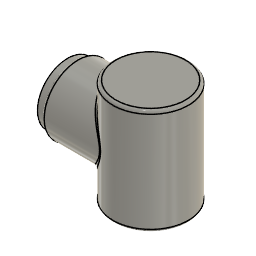
Assembly (Autodesk Fusion 360 archive; units mm, degrees)
design "link 04"
part number: 2026-05-23-14-39-53-080
Autodesk Fusion 360 part; units mm, degrees
note: some values were not read from the file. Set by a fixed rule: the direction of a hole.
sketch "Sketch1" plane through (0, 0, 0) normal (0, 0, 1) x (1, 0, 0)
  circle A0 centre (0, 0) radius 25
  dimension "d1" = 50
  constraint coincident A0.centre origin
  measures "d1" diameter of A0
extrude "Extrude1" add sketch "Sketch1" along normal blind 70
sketch "Sketch2" plane through (0, 0, 0) normal (1, 0, 0) x (0, 1, 0)
  circle A0 centre (0, 35) radius 22.5
  point P0 (0, 70)
  dimension "d4" = 45
  dimension "d5" = 35
  measures "d4" diameter of A0
  measures "d5" vertical distance of A0.centre P0
extrude "Extrude2" add sketch "Sketch2" against normal blind 50
sketch "Sketch3" plane through (-50, 0, 0) normal (-1, 0, 0) x (0, -1, 0)
sketch "Sketch4" plane through (-50, 0, 0) normal (-1, 0, 0) x (0, -1, 0)
sketch "Sketch5" plane through (-50, 0, 0) normal (-1, 0, 0) x (0, -1, 0)
  circle A0 centre (0, 35) radius 20
  dimension "d12" = 40
  measures "d12" diameter of A0
extrude "Extrude3" add sketch "Sketch5" along normal blind 5
fillet "Fillet3" radius 2 4 edges at (-23.3082, -9.0404, 70) (-23.3082, -9.0404, 0) (-10.8972, 22.5, 35) (-50, -20.9774, 43.1363)

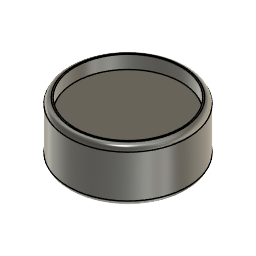
design "link 05"
part number: 2026-05-23-15-50-52-912
Autodesk Fusion 360 part; units mm, degrees
sketch "Sketch1" plane through (0, 0, 0) normal (0, 0, 1) x (1, 0, 0)
  circle A0 centre (0, 0) radius 22.5
  dimension "d1" = 45
  constraint coincident A0.centre origin
  measures "d1" diameter of A0
extrude "Extrude1" add sketch "Sketch1" along normal blind 20
sketch "Sketch2" plane through (0, 0, 20) normal (0, 0, 1) x (-1, 0, 0)
  circle A0 centre (0, 0) radius 22.5
  circle A1 centre (0, 0) radius 20
  dimension "d4" = 40
  constraint coincident A0.centre A1.centre
  measures "d4" diameter of A1
extrude "Extrude2" cut sketch "Sketch2" against normal blind 5 contours A1
sketch "Sketch3" plane through (0, 0, 0) normal (0, 0, 1) x (1, 0, 0)
  circle A0 centre (0, 0) radius 12.5
  dimension "d7" = 25
  constraint coincident A0.centre origin
  measures "d7" diameter of A0
extrude "Extrude3" cut sketch "Sketch3" along normal blind 5
sketch "Sketch4" plane through (0, 0, 0) normal (0, 0, -1) x (1, 0, 0)
  circle A0 centre (0, 0) radius 12.5
  circle A1 centre (0, 0) radius 22.5
  circle A2 centre (0, 0) radius 17.2047
  line L0 (0, 0) -> (-12, 12)
  line L1 (-12, 12) -> (0, 0)
  line L2 (0, 0) -> (12.1655, -12.1655)
  line L3 (0, 0) -> (12, 12)
  line L4 (12, 12) -> (0, 0)
  line L5 (0, 0) -> (-12, -12)
  point P0 (0, 17.2047)
  point P1 (12.1655, 12.1655)
  point P2 (17.2045, -0.0657)
  point P3 (12.1655, -12.1655)
  point P4 (-0.0267, -17.2046)
  point P5 (-12.1655, -12.1655)
  point P6 (-12, 12)
  point P7 (-17.2047, 0)
  constraint coincident A0.centre A1.centre
  constraint coincident A2 P0
  constraint coincident A2 P3
  constraint parallel L1 L2
  constraint perpendicular L2 L3
  constraint perpendicular L1 L5
  constraint coincident A2 P1
  constraint coincident A2 P2
  constraint coincident P3 L2.end
  constraint coincident A2 P4
  constraint coincident A2 P5
  constraint coincident P6 L0.end
  constraint coincident A2 P7
hole "Hole1" at (0, -17.2047, 0) at (-12, -12, 0) at (-17.2047, 0, 0) at (-12, 12, 0) at (-0.0267, 17.2046, 0) at (12.1655, 12.1655, 0) at (17.2045, 0.0657, 0) at (12.1655, -12.1655, 0) direction (0, 0, 1) diameter 5.035 depth 6 tip angle 118
thread "Thread1" "ISO Metric profile 6.0 M6x1 M6x1 6H" thread offset 0 thread depth 7.4
fillet "Fillet1" radius 2 1 edges at (-20.9774, -8.1363, 20) 1 faces at (-22.472, 1.1215, 6.6667)

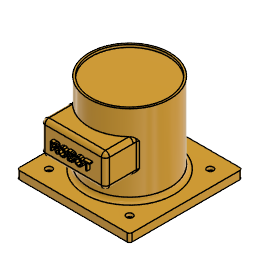
design "base"
part number: 2026-05-23-09-46-44-158
Autodesk Fusion 360 part; units mm, degrees
sketch "Sketch1" plane through (0, 0, 0) normal (0, 0, 1) x (1, 0, 0)
  line L0 (-70, 70) -> (70, 70)
  line L1 (70, 70) -> (70, -70)
  line L2 (70, -70) -> (-70, -70)
  line L3 (-70, -70) -> (-70, 70)
  constraint horizontal L0
  constraint vertical L1
  constraint horizontal L2
  constraint vertical L3
extrude "Extrude1" add sketch "Sketch1" along normal blind 10
sketch "Sketch2" plane through (0, 0, 10) normal (0, 0, 1) x (-1, 0, 0)
  line L0 (70, 70) -> (-70, 70)
  line L1 (-70, 70) -> (-70, -70)
  line L2 (-70, -70) -> (70, -70)
  line L3 (70, -70) -> (70, 70)
  circle A0 centre (0, 0) radius 50
  dimension "d3" = 100
  constraint coincident A0.centre origin
  measures "d3" diameter of A0
extrude "Extrude2" add sketch "Sketch2" along normal blind 100 contours A0
sketch "Sketch3" plane through (0, 0, 0) normal (0, 1, 0) x (1, 0, 0)
  line L0 (-40, -80) -> (40, -80)
  line L1 (40, -80) -> (40, -40)
  line L2 (40, -40) -> (-40, -40)
  line L3 (-40, -40) -> (-40, -80)
  dimension "d6" = 80
  dimension "d7" = 40
  dimension "d8" = 40
  dimension "d9" = 40
  constraint horizontal L0
  constraint vertical L1
  constraint horizontal L2
  constraint vertical L3
  measures "d6" distance of L0.start L0.end
  measures "d7" distance of L0.start L2.end
  measures "d8" horizontal distance of origin L2.end
  measures "d9" distance of origin L2
extrude "Extrude3" add sketch "Sketch3" against normal blind 70
sketch "Sketch4" plane through (0, 0, 110) normal (0, 0, 1) x (-1, 0, 0)
  circle A0 centre (0, 0) radius 50
  circle A1 centre (0, 0) radius 47.5
  dimension "d12" = 95
  constraint coincident A0.centre A1.centre
  measures "d12" diameter of A1
extrude "Extrude4" cut sketch "Sketch4" against normal blind 3 contours A1
sketch "Sketch5" plane through (0, 0, 10) normal (0, 0, 1) x (-1, 0, 0)
  circle A0 centre (0, 0) radius 50
  line L0 (70, 70) -> (-70, 70)
  line L1 (-70, 70) -> (-70, -70)
  line L2 (-70, -70) -> (70, -70)
  line L3 (70, -70) -> (70, 70)
  point P0 (50, -50)
  point P1 (-50, -50)
  point P2 (-50, 50)
  point P3 (50, 50)
  dimension "d15" = 20
  dimension "d16" = 20
  dimension "d17" = 20
  dimension "d18" = 20
  dimension "d19" = 20
  dimension "d20" = 20
  dimension "d21" = 20
  dimension "d22" = 20
  measures "d15" vertical distance of L2.end P0
  measures "d16" horizontal distance of L2.end P0
  measures "d17" vertical distance of L1.end P1
  measures "d18" horizontal distance of L1.end P1
  measures "d19" vertical distance of L0.end P2
  measures "d20" horizontal distance of L0.end P2
  measures "d21" vertical distance of L0.start P3
  measures "d22" horizontal distance of L0.start P3
hole "Hole1" at (50, 50, 10) at (-50, 50, 10) at (-50, -50, 10) at (50, -50, 10) direction (0, 0, -1) diameter 4.5 depth 40 tip angle 118 counterbore diameter 8 counterbore depth 4
fillet "Fillet1" radius 3 4 edges at (70, -70, 5) (-70, -70, 5) (70, 70, 5) (-70, 70, 5)
fillet "Fillet2" radius 5 4 edges at (40, -70, 60) (-40, -70, 60) (-40, -30, 60) (40, -30, 60)
fillet "Fillet3" radius 5 7 edges at (40.2327, -30.1152, 80) (40, -48.3114, 80) (38.5355, -68.5355, 80) (0, -70, 80) (-38.5355, -68.5355, 80) (-40, -48.3114, 80) (-40.2327, -30.1152, 80)
fillet "Fillet4" radius 5 7 edges at (-40.2327, -30.1152, 40) (-40, -48.3114, 40) (-38.5355, -68.5355, 40) (0, -70, 40) (38.5355, -68.5355, 40) (40, -48.3114, 40) (40.2327, -30.1152, 40)
fillet "Fillet5" radius 5 1 edges at (46.6164, -18.0808, 10)
sketch "Sketch7" plane through (0, -70, 0) normal (0, -1, 0) x (1, 0, 0)
  line L0 (-35, 45) -> (35, 45)
  line L1 (35, 45) -> (35, 75)
  line L2 (35, 75) -> (-35, 75)
  line L3 (-35, 75) -> (-35, 45)
  line L4 (-35, 45) -> (35, 45) construction
  line L5 (35, 45) -> (35, 75) construction
  line L6 (35, 75) -> (-35, 75) construction
  line L7 (-35, 75) -> (-35, 45) construction
  dimension "d44" = 10
  text T0 "ROBOT" font "Arial" height 10 align centre middle in box 70 x 30 at (-35, 45) x (1, 0) y (0, 1) spacing 1 kerned
  constraint coincident L0.end
  constraint coincident L2.end
extrude "Extrude6" add sketch "Sketch7" along normal blind 4 text T0
equation "d45 = 'ROBOT'"

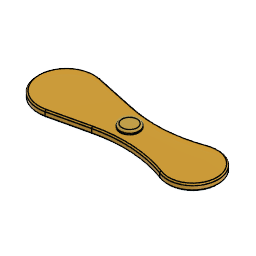
design "Link 01"
part number: 2026-05-23-11-57-22-292
Autodesk Fusion 360 part; units mm, degrees
sketch "Sketch1" plane through (0, 0, 0) normal (0, 0, 1) x (1, 0, 0)
  circle A0 centre (0, 0) radius 45
  circle A1 centre (200, 0) radius 40
  line L0 (9.3968, 44.008) -> (75, 30)
  arc A2 (75, 30) -> (188.4082, 38.2835) centre (117.4765, 228.9292) ccw
  line L1 (10.1387, -43.843) -> (70, -30)
  arc A3 (184.6116, -36.9215) -> (70, -30) centre (115.6051, -227.2104) ccw
  dimension "d1" = 90
  dimension "d2" = 80
  dimension "d3" = 200
  constraint coincident A0.centre origin
  constraint coincident A0 L0.start
  constraint tangent A0 L0
  constraint coincident A1 A2.end
  constraint tangent L0 A2
  constraint coincident A0 L1.start
  constraint tangent A0 L1
  constraint coincident A1 A3.start
  constraint tangent L1 A3
  measures "d1" diameter of A0
  measures "d2" diameter of A1
  measures "d3" distance of A0.centre A1.centre
extrude "Extrude1" add sketch "Sketch1" along normal blind 10
sketch "Sketch3" plane through (0, 0, 0) normal (0, 0, -1) x (1, 0, 0)
  arc A0 (10.1387, 43.843) -> (9.3968, -44.008) centre (0, 0) ccw
  line L0 (9.3968, -44.008) -> (75, -30)
  arc A1 (184.4992, -36.8744) -> (75, -30) centre (117.4765, -228.9292) ccw
  arc A2 (184.4992, -36.8744) -> (184.6116, 36.9215) centre (200, 0) ccw
  arc A3 (70, 30) -> (184.6116, 36.9215) centre (115.6051, 227.2104) ccw
  line L1 (70, 30) -> (10.1387, 43.843)
fillet "Fillet3" radius 2 12 edges at (130.2218, 25.9153, 10) (42.1984, 37.004, 10) (-44.9984, -0.38, 10) (40.0694, -36.9215, 10) (127.8069, -25.1637, 10) (240, 0.0609, 10) (240, 0.0609, 0) (127.8069, -25.1637, 0) (40.0694, -36.9215, 0) (-44.9984, -0.38, 0) (42.1984, 37.004, 0) (130.2218, 25.9153, 0)
sketch "Sketch4" plane through (0, 0, 10) normal (0, 0, 1) x (-1, 0, 0)
  arc A0 (-185.3383, 35.0576) -> (-185.2178, -35.0069) centre (-200, 0) ccw
  arc A1 (-74.5824, -28.0441) -> (-185.2178, -35.0069) centre (-117.4765, -228.9292) ccw
  line L0 (-74.5824, -28.0441) -> (-8.9792, -42.052)
  arc A2 (-8.9792, -42.052) -> (-9.6881, 41.8944) centre (0, 0) ccw
  line L1 (-9.6881, 41.8944) -> (-69.5494, 28.0514)
  arc A3 (-185.3383, 35.0576) -> (-69.5494, 28.0514) centre (-115.6051, 227.2104) ccw
  circle A4 centre (-100, 0) radius 15
  dimension "d22" = 30
  measures "d22" diameter of A4
extrude "Extrude2" add sketch "Sketch4" along normal blind 5 contours A4
sketch "Sketch5" plane through (0, 0, 15) normal (0, 0, 1) x (-1, 0, 0)
  circle A0 centre (-100, 0) radius 15
fillet "Fillet4" radius 3 1 faces at (105.2189, -1.9491, 15)

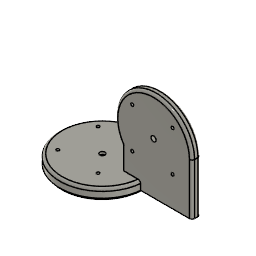
design "Link"
part number: 2026-05-23-10-24-38-964
Autodesk Fusion 360 part; units mm, degrees
sketch "Sketch1" plane through (0, 0, 0) normal (0, 0, 1) x (1, 0, 0)
sketch "Sketch2" plane through (0, 0, 0) normal (0, 0, 1) x (1, 0, 0)
sketch "Sketch3" plane through (0, 0, 0) normal (0, 0, 1) x (1, 0, 0)
sketch "Sketch4" plane through (0, 0, 0) normal (0, 0, 1) x (1, 0, 0)
  circle A0 centre (0, 0) radius 50
  dimension "d1" = 100
  constraint coincident A0.centre origin
  measures "d1" diameter of A0
extrude "Extrude1" add sketch "Sketch4" along normal blind 10
sketch "Sketch5" plane through (0, 0, 0) normal (0, 0, 1) x (1, 0, 0)
  circle A0 centre (0, 0) radius 47.5
  dimension "d4" = 95
  constraint coincident A0.centre origin
  measures "d4" diameter of A0
extrude "Extrude2" add sketch "Sketch5" against normal blind 3
sketch "Sketch6" plane through (0, 0, 0) normal (0, 1, 0) x (1, 0, 0)
  line L0 (30, 0) -> (110, 0)
  line L1 (110, 0) -> (110, -50)
  line L2 (110, -50) -> (110, -60)
  arc A0 (30, -31.7157) -> (110, -60) centre (65, -60) ccw
  line L3 (30, -31.7157) -> (30, 0)
  dimension "d7" = 80
  dimension "d8" = 50
  dimension "d9" = 45
  dimension "d10" = 30
  dimension "d11" = 60
  constraint horizontal L0
  constraint perpendicular L0 L1
  constraint parallel L1 L2
  constraint tangent L2 A0
  constraint perpendicular L0 L3
  measures "d7" distance of L0.start L0.end
  measures "d8" distance of L0.end L1.end
  measures "d9" radius of A0
  measures "d10" distance of origin L0.start
  measures "d11" vertical distance of origin A0.centre
extrude "Extrude3" add sketch "Sketch6" along normal mid plane 10
sketch "Sketch7" plane through (0, 5, 0) normal (0, 1, 0) x (-1, 0, 0)
  line L0 (-49.7494, 10) -> (-30, 10)
  line L1 (-30, 10) -> (-30, 31.7157)
  arc A0 (-30, 31.7157) -> (-110, 60) centre (-65, 60) ccw
  line L2 (-110, 60) -> (-110, 0)
  line L3 (-110, 0) -> (-49.7494, 0)
  line L4 (-49.7494, 0) -> (-49.7494, 10)
  line L5 (-87.244, 82.244) -> (-40, 82.244)
  line L6 (-40, 82.244) -> (-40, 35)
  line L7 (-40, 35) -> (-87.244, 35)
  line L8 (-87.244, 35) -> (-87.244, 82.244)
  dimension "d14" = 47.244
  dimension "d15" = 47.244
  dimension "d16" = 25
  dimension "d17" = 25
  constraint horizontal L5
  constraint vertical L6
  constraint horizontal L7
  constraint vertical L8
  measures "d14" distance of L5.start L5.end
  measures "d15" distance of L5.start L7.end
  measures "d16" vertical distance of A0.centre L7.end
  measures "d17" horizontal distance of A0.centre L6.end
hole "Hole1" at (40, 5, 82.244) at (87.244, 5, 82.244) at (87.244, 5, 35) at (40, 5, 35) direction (0, -1, 0) diameter 3.332 end through all
thread "Thread2" "ISO Metric profile 4.0 M4x0.7 M4x0.7 6H" major diameter 4.1095 minor diameter 3.332 pitch 0.7 angle 60 resizes the face on face at (39.2032, 1.6667, 33.5369) on face at (88.4931, 1.6667, 33.8976) on face at (38.3345, 1.6667, 82.2025) on face at (85.9949, 1.6667, 83.3464)
hole "Hole2" at (65, 5, 60) direction (0, -1, 0) diameter 6 end through all
sketch "Sketch8" plane through (0, 0, 10) normal (0, 0, 1) x (-1, 0, 0)
  line L0 (-30, -5) -> (-49.7494, -5)
  arc A0 (-49.7494, -5) -> (-49.7494, 5) centre (0, 0) ccw
  line L1 (-49.7494, 5) -> (-30, 5)
  line L2 (-30, 5) -> (-30, -5)
  line L3 (30, -25) -> (-17.244, -25)
  line L4 (-17.244, -25) -> (-17.244, 22.244)
  line L5 (-17.244, 22.244) -> (30, 22.244)
  line L6 (30, 22.244) -> (30, -25)
  dimension "d22" = 47.244
  dimension "d23" = 47.244
  dimension "d24" = 30
  dimension "d25" = 25
  constraint horizontal L3
  constraint vertical L4
  constraint horizontal L5
  constraint vertical L6
  measures "d22" distance of L3.start L3.end
  measures "d23" distance of L3.start L5.end
  measures "d24" horizontal distance of A0.centre L3.start
  measures "d25" vertical distance of A0.centre L3.end
hole "Hole3" at (-30, 25, 10) at (17.244, 25, 10) at (17.244, -22.244, 10) at (-30, -22.244, 10) direction (0, 0, -1) diameter 3.332 depth 10 tip angle 118
thread "Thread1" "ISO Metric profile 4.0 M4x0.7 M4x0.7 6H" major diameter 4.1095 minor diameter 3.332 pitch 0.7 angle 60 resizes the face on face at (16.1731, 26.2762, 6.6667) on face at (16.1731, -20.9678, 6.6667) on face at (-31.0709, -20.9678, 6.6667) on face at (-31.0709, 26.2762, 6.6667)
hole "Hole4" at (0, 0, 0) direction (0, 0, -1) diameter 6 end through all
hole "Hole5" at (0, 0, 0) direction (0, 0, 1) diameter 6 depth 3 tip angle 118
sketch "Sketch9" plane through (0, 0, 10) normal (0, 0, 1) x (-1, 0, 0)
  circle A0 centre (-17.244, 22.244) radius 1.666
  circle A1 centre (30, -25) radius 1.666
  circle A2 centre (-17.244, -25) radius 1.666
  circle A3 centre (30, 22.244) radius 1.666
  line L0 (-30, -5) -> (-49.7494, -5)
  arc A4 (-49.7494, -5) -> (-49.7494, 5) centre (0, 0) ccw
  line L1 (-49.7494, 5) -> (-30, 5)
  line L2 (-30, 5) -> (-30, -5)
hole "Hole6" at (0, 0, 10) direction (0, 0, -1) diameter 6 depth 3 tip angle 118
fillet "Fillet1" radius 3 1 edges at (-50, 0, 10)
fillet "Fillet2" radius 3 4 edges at (110, -5, 30) (50, -5, 102.4264) (50, 5, 102.4264) (110, 5, 30)

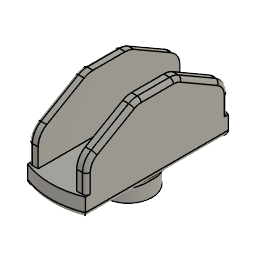
design "link 07"
part number: 2026-05-24-12-09-00-138
Autodesk Fusion 360 part; units mm, degrees
sketch "Sketch1" plane through (0, 0, 0) normal (0, 0, 1) x (1, 0, 0)
  circle A0 centre (0, 0) radius 12.5
  dimension "d1" = 25
  constraint coincident A0.centre origin
  measures "d1" diameter of A0
extrude "Extrude1" add sketch "Sketch1" along normal blind 10
sketch "Sketch2" plane through (0, 0, 10) normal (0, 0, 1) x (-1, 0, 0)
  circle A0 centre (0, 0) radius 12.5
  circle A1 centre (0, 0) radius 40
  dimension "d4" = 80
  constraint coincident A0.centre A1.centre
  measures "d4" diameter of A1
extrude "Extrude2" add sketch "Sketch2" along normal blind 10 contours A0 | A1
sketch "Sketch7" plane through (0, 0, 20) normal (0, 0, 1) x (-1, 0, 0)
  circle A0 centre (0, 0) radius 40
  line L0 (-15, -40) -> (-64.6051, -40)
  line L1 (-64.6051, -40) -> (-64.6051, 41.753)
  line L2 (-64.6051, 41.753) -> (-15, 41.753)
  line L3 (-15, 41.753) -> (-15, -40)
  dimension "d40" = 81.753
  dimension "d41" = 15
  constraint horizontal L0
  constraint vertical L1
  constraint horizontal L2
  constraint vertical L3
  measures "d40" distance of L0.start L2.end
  measures "d41" horizontal distance of A0.centre L0.start
extrude "Extrude7" cut sketch "Sketch7" against normal blind 10 contours A0 L3 picked at (-23.3333, 0)
mirror "Mirror3" about plane through (0, 0, 0) normal (1, 0, 0) of "Extrude7"
sketch "Sketch8" plane through (0, 0, 20) normal (0, 0, 1) x (-1, 0, 0)
  line L0 (15, -37.081) -> (15, 37.081)
  arc A0 (15, 37.081) -> (-15, 37.081) centre (0, 0) ccw
  line L1 (-15, 37.081) -> (-15, -37.081)
  arc A1 (-15, -37.081) -> (15, -37.081) centre (0, 0) ccw
  line L2 (-10, -36.9362) -> (-15, -36.9362)
  line L3 (-15, -36.9362) -> (-15, 36.6135)
  line L4 (-15, 36.6135) -> (-10, 36.6135)
  line L5 (-10, 36.6135) -> (-10, -36.9362)
  dimension "d67" = 5
  dimension "d68" = 10
  constraint horizontal L2
  constraint vertical L3
  constraint horizontal L4
  constraint vertical L5
  measures "d67" distance of L2.start L2.end
  measures "d68" horizontal distance of A0.centre L2.start
extrude "Extrude8" add sketch "Sketch8" along normal blind 30 contours L1 L2 L3 L4 L5
sketch "Sketch9" plane through (15, 0, 0) normal (1, 0, 0) x (0, 1, 0)
  line L0 (-36.6135, 20) -> (-37.081, 20)
  line L1 (-37.081, 20) -> (-37.081, 10)
  line L2 (-37.081, 10) -> (37.081, 10)
  line L3 (37.081, 10) -> (37.081, 20)
  line L4 (37.081, 20) -> (36.9362, 20)
  line L5 (36.9362, 20) -> (36.9362, 50)
  line L6 (36.9362, 50) -> (-36.6135, 50)
  line L7 (-36.6135, 50) -> (-36.6135, 20)
  line L8 (-36.6135, 35) -> (-10.1568, 50.2748)
  line L9 (-36.6135, 35) -> (-6.0639, 35) construction
  line L10 (36.9362, 35) -> (10.9555, 50)
  line L11 (36.9362, 35) -> (66.9362, 35) construction
  dimension "d49" = 30
  dimension "d50" = 150
  constraint horizontal L9
  constraint midpoint L7 L8.start
  constraint horizontal L11
  constraint midpoint L5 L10.start
  constraint coincident L6 L10.end
  measures "d49" angle of L8 L9
  measures "d50" angle of L10 L11
extrude "Extrude9" cut sketch "Sketch9" against normal blind 10 contours L6 L7 L8 | L5 L6 L10
fillet "Fillet7" radius 9 4 edges at (12.5, 10.9555, 50) (12.5, -10.6328, 50) (12.5, -36.6135, 35) (12.5, 36.9362, 35)
fillet "Fillet8" radius 2 9 edges at (15, -36.6135, 24.9019) (15, -35.4077, 34.3038) (15, -22.4174, 43.1962) (15, -10.5506, 49.6933) (15, 0.1614, 50) (15, 10.8733, 49.6933) (15, 22.7401, 43.1962) (15, 35.7305, 34.3038) (15, 36.9362, 24.9019)
fillet "Fillet9" radius 3 1 edges at (15, -37.081, 15)
fillet "Fillet10" radius 3 1 edges at (15, 37.081, 15)
fillet "Fillet11" radius 3 1 faces at (8.4107, -28.8289, 10)
mirror "Mirror4" about plane through (0, 0, 0) normal (1, 0, 0) of bodies 1 merged

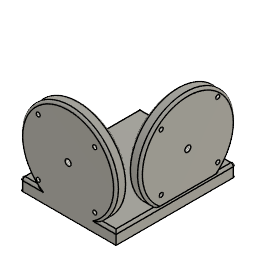
design "link 02"
part number: 2026-05-23-12-24-57-202
Autodesk Fusion 360 part; units mm, degrees
sketch "Sketch1" plane through (0, 0, 0) normal (0, 0, 1) x (1, 0, 0)
  line L0 (0, 0) -> (80, 0)
  line L1 (80, 0) -> (80, 100)
  line L2 (80, 100) -> (0, 100)
  line L3 (0, 100) -> (0, 0)
  dimension "d1" = 80
  dimension "d2" = 100
  constraint horizontal L0
  constraint vertical L1
  constraint horizontal L2
  constraint vertical L3
  constraint coincident L0.start L3.end
  measures "d1" distance of L0.start L0.end
  measures "d2" distance of L0.start L2.end
extrude "Extrude1" add sketch "Sketch1" along normal blind 10 makes body 1
sketch "Sketch2" plane through (0, 0, 0) normal (0, 1, 0) x (1, 0, 0)
  circle A0 centre (40, -40) radius 40
  line L0 (0, 0) -> (80, 0)
  dimension "d5" = 80
  dimension "d6" = 40
  dimension "d7" = 40
  measures "d5" diameter of A0
  measures "d6" horizontal distance of L0.start A0.centre
  measures "d7" distance of A0.centre L0
extrude "Extrude2" add sketch "Sketch2" along normal blind 10 bodies 1
sketch "Sketch3" plane through (80, 0, 0) normal (1, 0, 0) x (0, 1, 0)
  line L0 (0, 0) -> (100, 0)
  line L1 (100, 0) -> (100, 10)
  line L2 (100, 10) -> (0, 10)
  line L3 (0, 10) -> (0, 0)
  circle A0 centre (60, 40) radius 40
  dimension "d10" = 80
  dimension "d11" = 40
  dimension "d12" = 60
  measures "d10" diameter of A0
  measures "d11" distance of L0 A0.centre
  measures "d12" horizontal distance of L0.start A0.centre
extrude "Extrude3" add sketch "Sketch3" against normal blind 10 separate body contours L2 A0 picked at (48.0445, 46.6728) makes body 2
sketch "Sketch4" plane through (0, 10, 0) normal (0, 1, 0) x (-1, 0, 0)
  line L0 (-66.4575, 10) -> (-13.5425, 10)
  arc A0 (-13.5425, 10) -> (-66.4575, 10) centre (-40, 40) ccw
  line L1 (-62.244, 62.244) -> (-15, 62.244)
  line L2 (-15, 62.244) -> (-15, 15)
  line L3 (-15, 15) -> (-62.244, 15)
  line L4 (-62.244, 15) -> (-62.244, 62.244)
  dimension "d19" = 47.244
  dimension "d20" = 47.244
  dimension "d21" = 25
  dimension "d22" = 25
  constraint horizontal L1
  constraint vertical L2
  constraint horizontal L3
  constraint vertical L4
  measures "d19" distance of L1.start L1.end
  measures "d20" distance of L1.start L3.end
  measures "d21" vertical distance of A0.centre L2.end
  measures "d22" horizontal distance of A0.centre L1.end
hole "Hole1" at (62.244, 10, 62.244) at (15, 10, 62.244) at (15, 10, 15) at (62.244, 10, 15) direction (0, -1, 0) diameter 3.332 end through all bodies 1
thread "Thread1" "ISO Metric profile 4.0 M4x0.7 M4x0.7 6H" major diameter 4.1095 minor diameter 3.332 pitch 0.7 angle 60 resizes the face on face at (15.083, 6.6667, 16.6639) on face at (15.083, 6.6667, 63.9079) on face at (61.6742, 6.6667, 16.5655) on face at (61.4472, 6.6667, 60.7809) on bodies 1
sketch "Sketch5" plane through (70, 0, 0) normal (-1, 0, 0) x (0, -1, 0)
  arc A0 (-33.5425, 10) -> (-86.4575, 10) centre (-60, 40) ccw
  line L0 (-86.4575, 10) -> (-33.5425, 10)
  line L1 (-85, 65) -> (-37.756, 65)
  line L2 (-37.756, 65) -> (-37.756, 17.756)
  line L3 (-37.756, 17.756) -> (-85, 17.756)
  line L4 (-85, 17.756) -> (-85, 65)
  dimension "d27" = 47.244
  dimension "d28" = 47.244
  dimension "d29" = 25
  dimension "d30" = 25
  constraint horizontal L1
  constraint vertical L2
  constraint horizontal L3
  constraint vertical L4
  measures "d27" distance of L1.start L1.end
  measures "d28" distance of L1.start L3.end
  measures "d29" horizontal distance of A0.centre L1.start
  measures "d30" vertical distance of A0.centre L1.end
hole "Hole2" at (70, 37.756, 65) at (70, 85, 65) at (70, 85, 17.756) at (70, 37.756, 17.756) direction (1, 0, 0) diameter 3.332 depth 10 tip angle 118 bodies 2
thread "Thread2" "ISO Metric profile 4.0 M4x0.7 M4x0.7 6H" major diameter 4.1095 minor diameter 3.332 pitch 0.7 angle 60 resizes the face on face at (73.3333, 83.7509, 66.1024) on face at (73.3333, 37.1862, 19.3215) on face at (73.3333, 36.0905, 64.9585) on face at (73.3333, 86.0709, 16.4798) on bodies 2
sketch "Sketch6" plane through (0, 0, 0) normal (0, -1, 0) x (1, 0, 0)
  circle A0 centre (15, 15) radius 1.666
  circle A1 centre (62.244, 62.244) radius 1.666
  circle A2 centre (15, 62.244) radius 1.666
  circle A3 centre (62.244, 15) radius 1.666
  line L0 (13.5425, 10) -> (0, 10)
  line L1 (0, 10) -> (0, 0)
  line L2 (0, 0) -> (80, 0)
  line L3 (80, 0) -> (80, 10)
  line L4 (80, 10) -> (66.4575, 10)
  arc A4 (66.4575, 10) -> (13.5425, 10) centre (40, 40) ccw
hole "Hole3" at (40, 0, 40) direction (0, 1, 0) diameter 5.035 depth 10 tip angle 118 bodies 1
thread "Thread3" "ISO Metric profile 6.0 M6x1 M6x1 6H" major diameter 6.147 minor diameter 5.035 pitch 1 angle 60 resizes the face on face at (40.1255, 3.3333, 37.4856) on bodies 1
sketch "Sketch7" plane through (80, 0, 0) normal (1, 0, 0) x (0, 1, 0)
  circle A0 centre (85, 17.756) radius 1.666
  circle A1 centre (37.756, 65) radius 1.666
  circle A2 centre (85, 65) radius 1.666
  circle A3 centre (37.756, 17.756) radius 1.666
  arc A4 (86.4575, 10) -> (33.5425, 10) centre (60, 40) ccw
  line L0 (33.5425, 10) -> (86.4575, 10)
hole "Hole4" at (80, 60, 40) direction (-1, 0, 0) diameter 5.035 end through all bodies 2
thread "Thread4" "ISO Metric profile 6.0 M6x1 M6x1 6H" major diameter 6.147 minor diameter 5.035 pitch 1 angle 60 resizes the face on face at (76.6667, 60.1255, 37.4856) on bodies 2
fillet "Fillet1" radius 2 2 edges at (40, 100, 10) (0, 50, 10) on bodies 1
fillet "Fillet2" radius 2 4 edges at (80, 49, 10) (80, 99.4142, 9.4142) (80, 100, 4) (73.2288, 0, 10) on bodies 1
fillet "Fillet3" radius 2 4 edges at (0, 0, 4) (0.5858, 0, 9.4142) (7.7712, 0, 10) (41.5842, 0, 79.9686) on bodies 1
fillet "Fillet4" radius 2 1 edges at (40, 10, 80) on bodies 1
fillet "Fillet5" radius 2 2 edges at (70, 60, 80) (80, 60, 80) on bodies 2

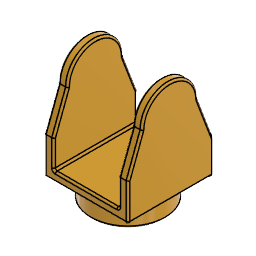
design "link 03"
part number: 2026-05-23-13-09-46-882
Autodesk Fusion 360 part; units mm, degrees
sketch "Sketch1" plane through (0, 0, 0) normal (0, 0, 1) x (1, 0, 0)
  line L0 (0, 0) -> (90, 0)
  line L1 (90, 0) -> (90, 90)
  line L2 (90, 90) -> (0, 90)
  line L3 (0, 90) -> (0, 0)
  dimension "d1" = 90
  dimension "d2" = 90
  constraint horizontal L0
  constraint vertical L1
  constraint horizontal L2
  constraint vertical L3
  constraint coincident L0.start L3.end
  measures "d1" distance of L0.start L0.end
  measures "d2" distance of L0.start L2.end
extrude "Extrude1" add sketch "Sketch1" along normal blind 10
sketch "Sketch2" plane through (0, 0, 0) normal (0, 0, -1) x (1, 0, 0)
  line L0 (0, 0) -> (0, -90)
  line L1 (0, -90) -> (90, -90)
  line L2 (90, -90) -> (90, 0)
  line L3 (90, 0) -> (0, 0)
  circle A0 centre (45, -45) radius 40
  dimension "d5" = 80
  dimension "d6" = 45
  dimension "d7" = 45
  measures "d5" diameter of A0
  measures "d6" vertical distance of L2.end A0.centre
  measures "d7" horizontal distance of L1.end A0.centre
extrude "Extrude2" add sketch "Sketch2" along normal blind 20 contours A0
fillet "Fillet1" radius 2 1 edges at (7.7069, 59.4646, -20)
sketch "Sketch3" plane through (90, 0, 0) normal (1, 0, 0) x (0, 1, 0)
  line L0 (0, 0) -> (90, 0)
  line L1 (90, 0) -> (90, 10)
  line L2 (90, 10) -> (0, 10)
  line L3 (0, 10) -> (0, 0)
  line L4 (0, 0) -> (90, 0)
  line L5 (90, 0) -> (90, 40)
  line L6 (90, 40) -> (0, 40)
  line L7 (0, 40) -> (0, 0)
  circle A0 centre (45, 80) radius 30
  line L8 (15.0001, 79.9162) -> (0, 40)
  line L9 (74.9999, 79.9162) -> (90, 40)
  dimension "d12" = 40
  dimension "d13" = 60
  dimension "d14" = 45
  dimension "d15" = 80
  constraint horizontal L4
  constraint vertical L5
  constraint horizontal L6
  constraint vertical L7
  constraint coincident L0.start L3.end
  constraint coincident A0 L8.start
  constraint coincident A0 L9.start
  measures "d12" distance of L0.start L6.end
  measures "d13" diameter of A0
  measures "d14" horizontal distance of L0.start A0.centre
  measures "d15" vertical distance of L0.start A0.centre
extrude "Extrude3" add sketch "Sketch3" against normal blind 10 contours L2 L5 L6 L7 | L6 A0 L8 L9 | A0
sketch "Sketch4" plane through (0, 0, 0) normal (-1, 0, 0) x (0, -1, 0)
  line L0 (-90, 0) -> (0, 0)
  line L1 (0, 0) -> (0, 10)
  line L2 (0, 10) -> (-90, 10)
  line L3 (-90, 10) -> (-90, 0)
  line L4 (-90, 40) -> (0, 40)
  line L5 (0, 40) -> (0, 0)
  line L6 (0, 0) -> (-90, 0)
  line L7 (-90, 0) -> (-90, 40)
  circle A0 centre (-45, 80) radius 30
  line L8 (-90, 40) -> (-74.9982, 79.6754)
  line L9 (-15.0018, 79.6754) -> (0, 40)
  dimension "d18" = 60
  dimension "d19" = 80
  dimension "d20" = 45
  constraint horizontal L4
  constraint vertical L5
  constraint horizontal L6
  constraint vertical L7
  constraint coincident L0.end L1.start
  constraint coincident A0 L8.end
  constraint coincident A0 L9.start
  measures "d18" diameter of A0
  measures "d19" vertical distance of L0.end A0.centre
  measures "d20" horizontal distance of L0.end A0.centre
extrude "Extrude4" add sketch "Sketch4" against normal blind 10 contours L2 L4 L5 L7 | L4 A0 L8 L9 | A0
fillet "Fillet2" radius 2 26 edges at (10, 7.5009, 59.8377) (10, 0, 25) (45, 0, 10) (80, 0, 25) (80, 7.5001, 59.9581) (80, 45, 110) (10, 45, 110) (0, 45, 110) (0, 7.5009, 59.8377) (0, 0, 20) (45, 0, 0) (90, 45, 0) (80, 45, 10) (80, 90, 25) (80, 82.4999, 59.9581) (90, 82.4999, 59.9581) (90, 45, 110) (90, 7.5001, 59.9581) (90, 0, 20) (10, 82.4991, 59.8377) (0, 82.4991, 59.8377) (0, 90, 20) (10, 90, 25) (45, 90, 10) (45, 90, 0) (10, 45, 10)
fillet "Fillet3" radius 2 1 edges at (7.7069, 30.5354, 0)
